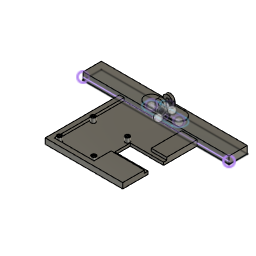
Plate (Autodesk Fusion 360 design; units mm, degrees)
Autodesk Fusion 360 part; units mm, degrees
sketch "스케치3" plane through (0, 0, 0) normal (0, 0, 1) x (1, 0, 0)
  line L0 (-80, 10) -> (80, 10)
  line L1 (80, 10) -> (80, -10)
  line L2 (80, -10) -> (-80, -10)
  line L3 (-80, -10) -> (-80, 10)
  dimension "d22" = 20
  dimension "d23" = 160
  dimension "d24" = 80
  dimension "d25" = 10
  constraint horizontal L0
  constraint vertical L1
  constraint horizontal L2
  constraint vertical L3
  measures "d22" distance of L0.end L1.end
  measures "d23" distance of L0.start L0.end
  measures "d24" distance of origin L1
  measures "d25" distance of origin L0
extrude "돌출3" add sketch "스케치3" along normal blind 3 and the other way blind 5
sketch "스케치4" plane through (0, 0, 3) normal (0, 0, 1) x (-1, 0, 0)
  arc A0 (-15, 7.5) -> (-15, -7.5) centre (-15, 0) ccw
  line L0 (0, 7.5) -> (-15, 7.5)
  line L1 (-15, -7.5) -> (0, -7.5)
  line L2 (80, 10) -> (-80, 10)
  line L3 (0, 7.5) -> (15, 7.5)
  arc A1 (15, -7.5) -> (15, 7.5) centre (15, 0) ccw
  line L4 (15, -7.5) -> (0, -7.5)
  dimension "d43" = 15
  measures "d43" distance of L0.start L1.end
extrude "돌출4" add sketch "스케치4" along normal blind 1
sketch "스케치6" plane through (0, 0, 0) normal (0, 1, 0) x (1, 0, 0)
  line L0 (-15, -4) -> (15, -4)
  line L1 (0, -4) -> (5, -4)
  line L2 (5, -4) -> (5, -10)
  line L3 (0, -4) -> (-3, -4)
  line L4 (-5, -10) -> (-5, -4)
  arc A0 (-5, -10) -> (5, -10) centre (0, -10) ccw
  line L5 (5, -4) -> (-5, -4)
  dimension "d34" = 5
  dimension "d68" = 6
  constraint midpoint L0 L1.start
  constraint parallel L0 L1
  constraint perpendicular L1 L2
  constraint coincident L0 L3.end
  constraint tangent L2 A0
  constraint coincident L0 L4.end
  constraint tangent L4 A0
  constraint perpendicular L0 L4
  measures "d34" distance of L1.start L1.end
  measures "d68" distance of L4.start L4.end
extrude "돌출5" add sketch "스케치6" along normal blind 3 from surface at 2.5
extrude "돌출6" add 1 faces at (1.6667, 2.5, 8) along direction (0, -1, 0) blind 3 from surface at 5.5
sketch "스케치7" plane through (0, 5.5, 0) normal (0, 1, 0) x (-1, 0, 0)
  circle A0 centre (0, 10) radius 1.7
  point P0 (0, 10)
  dimension "d41" = 3.4
  constraint coincident P0 A0.centre
  measures "d41" diameter of A0
extrude "돌출7" cut sketch "스케치7" against normal through all
move_body "이동1" bodies 1 to x (1, 0, 0) y (0, 1, 0) z (0, 0, 1) at (0, 0, 5)
sketch "스케치9" plane through (0, 0, 0) normal (0, 0, 1) x (1, 0, 0)
  line L0 (-80, -10) -> (80, -10)
  line L1 (-35, -10) -> (-35, -86.6)
  line L2 (-35, -86.6) -> (40, -86.6)
  line L3 (40, -86.6) -> (40, -10)
  line L4 (-35, -10) -> (40, -10)
  line L5 (-35, -10) -> (8.3, -10)
  line L6 (40, -67.8) -> (8.5, -67.8)
  line L7 (8.5, -67.8) -> (8.5, -86.6)
  line L8 (40, -43.3) -> (28, -43.3)
  line L9 (28, -43.3) -> (28, -10)
  dimension "d46" = 76.6
  dimension "d47" = 75
  dimension "d69" = 31.5
  dimension "d70" = 57.8
  dimension "d75" = 12
  dimension "d76" = 33.3
  constraint coincident L0 L1.start
  constraint perpendicular L0 L1
  constraint perpendicular L1 L2
  constraint coincident L0 L3.end
  constraint perpendicular L0 L3
  constraint perpendicular L1 L5
  constraint coincident L3 L6.start
  constraint perpendicular L3 L6
  constraint coincident L2 L7.end
  constraint perpendicular L2 L7
  constraint coincident L3 L8.start
  constraint perpendicular L3 L8
  constraint perpendicular L0 L9
  constraint coincident L0 L9.end
  measures "d46" distance of L1.start L1.end
  measures "d47" distance of L1.end L2.end
  measures "d69" distance of L6.start L6.end
  measures "d70" distance of L3.end L6.start
  measures "d75" distance of L8.start L8.end
  measures "d76" distance of L8.end L9.end
extrude "돌출8" add sketch "스케치9" along normal blind 3
sketch "스케치10" plane through (0, 0, 0) normal (0, 0, 1) x (1, 0, 0)
  line L0 (-40, -10) -> (-40, -91.6)
  line L1 (-40, -91.6) -> (45, -91.6)
  line L2 (45, -91.6) -> (45, -10)
  line L3 (-35, -10) -> (-35, -86.6)
  line L4 (-35, -86.6) -> (40, -86.6)
  line L5 (40, -86.6) -> (40, -10)
  line L6 (-35, -10) -> (-80, -10)
  line L7 (80, -10) -> (40, -10)
  dimension "d57" = 5
  dimension "d58" = 5
  dimension "d59" = 5
  constraint vertical L0
  constraint perpendicular L0 L1
  constraint perpendicular L1 L2
  constraint coincident L0.start L6
  constraint coincident L2.end L7
  measures "d57" distance of L0 L3
  measures "d58" distance of L1 L4
  measures "d59" distance of L2 L5
extrude "돌출9" add sketch "스케치10" sketch "스케치9" along normal blind 6 of sketch 2 contours L0 L3 L4 L8 L9 | L2 L3 L6 L7
sketch "스케치11" plane through (45, 0, 0) normal (1, 0, 0) x (0, 1, 0)
  line L0 (-86.6, 6) -> (-10, 6)
  line L1 (-10, 0) -> (-91.6, 0)
  line L2 (-67.8, 8) -> (-43.3, 8)
  line L3 (-43.3, 8) -> (-43.3, 3)
  line L4 (-43.3, 3) -> (-67.8, 3)
  line L5 (-67.8, 3) -> (-67.8, 8)
  point P0 (-67.8, 3)
  point P1 (-67.8, 6)
  point P2 (-43.3, 6)
  point P3 (-43.3, 3)
  dimension "d71" = 24.5
  dimension "d72" = 5
  constraint parallel L0 L2
  constraint perpendicular L2 L3
  constraint coincident P0 L4.end
  measures "d71" distance of L2.start L2.end
  measures "d72" distance of L2.end P3
extrude "돌출12" cut sketch "스케치11" against normal blind 5 contours L0 L3 L4 L5
sketch "스케치12" plane through (0, 0, 3) normal (0, 0, 1) x (-1, 0, 0)
  circle A0 centre (32.2, 83.8) radius 2.5
  line L0 (-8.5, 86.6) -> (35, 86.6)
  line L1 (35, 86.6) -> (35, 10)
  circle A1 centre (-5.5, 83.8) radius 2.5
  circle A2 centre (32.2, 46.8) radius 2.5
  circle A3 centre (-5.5, 46.8) radius 2.5
  dimension "d77" = 5
  dimension "d78" = 2.8
  dimension "d79" = 2.8
  dimension "d80" = 5
  dimension "d81" = 37.7
  dimension "d82" = 5
  dimension "d83" = 37
  dimension "d84" = 5
  measures "d77" diameter of A0
  measures "d78" distance of A0.centre L0
  measures "d79" distance of A0.centre L1
  measures "d80" diameter of A1
  measures "d81" distance of A0.centre A1.centre
  measures "d82" diameter of A2
  measures "d83" distance of A0.centre A2.centre
  measures "d84" diameter of A3
extrude "돌출13" add sketch "스케치12" along normal blind 5
sketch "스케치13" plane through (0, 0, 8) normal (0, 0, 1) x (-1, 0, 0)
  circle A0 centre (32.2, 46.8) radius 1.8
  circle A1 centre (32.2, 46.8) radius 2.5
  circle A2 centre (-5.5, 46.8) radius 1.8
  circle A3 centre (-5.5, 46.8) radius 2.5
  circle A4 centre (-5.5, 83.8) radius 1.8
  circle A5 centre (-5.5, 83.8) radius 2.5
  circle A6 centre (32.2, 83.8) radius 1.8
  circle A7 centre (32.2, 83.8) radius 2.5
  dimension "d87" = 3.6
  dimension "d88" = 3.6
  dimension "d89" = 3.6
  dimension "d90" = 3.6
  constraint concentric A0 A1
  constraint concentric A2 A3
  constraint concentric A4 A5
  constraint concentric A6 A7
  measures "d87" diameter of A0
  measures "d88" diameter of A2
  measures "d89" diameter of A4
  measures "d90" diameter of A6
extrude "돌출14" cut sketch "스케치13" against normal blind 1 contours A0 | A2 | A4 | A6
sketch "스케치14" plane through (0, 0, 7) normal (0, 0, 1) x (-1, 0, 0)
  circle A0 centre (32.2, 46.8) radius 1.25
  circle A1 centre (32.2, 46.8) radius 2.5
  circle A2 centre (-5.5, 46.8) radius 1.25
  circle A3 centre (-5.5, 46.8) radius 2.5
  circle A4 centre (-5.5, 83.8) radius 1.25
  circle A5 centre (-5.5, 83.8) radius 2.5
  circle A6 centre (32.2, 83.8) radius 1.25
  circle A7 centre (32.2, 83.8) radius 2.5
  dimension "d93" = 2.5
  dimension "d94" = 2.5
  dimension "d95" = 2.5
  dimension "d96" = 2.5
  constraint concentric A0 A1
  constraint concentric A2 A3
  constraint concentric A4 A5
  constraint concentric A6 A7
  measures "d93" diameter of A0
  measures "d94" diameter of A2
  measures "d95" diameter of A4
  measures "d96" diameter of A6
extrude "돌출15" cut sketch "스케치14" against normal blind 2 contours A0 | A2 | A4 | A6
sketch "스케치15" plane through (0, 0, 3) normal (0, 0, 1) x (-1, 0, 0)
  line L0 (-45, 63.8) -> (-8.5, 63.8)
  line L1 (-8.5, 63.8) -> (-8.5, 46.8)
  line L2 (-8.5, 46.8) -> (-45, 46.8)
  line L3 (-45, 46.8) -> (-45, 63.8)
  line L4 (-45, 43.3) -> (-45, 67.8)
  line L5 (-8.5, 67.8) -> (-8.5, 86.6)
  dimension "d99" = 17
  constraint horizontal L0
  constraint vertical L1
  constraint horizontal L2
  constraint vertical L3
  constraint coincident L0.start L4
  constraint collinear L1 L5
  measures "d99" distance of L0.start L2.end
extrude "돌출16" cut sketch "스케치15" against normal through all
equation "d46 = 43.3 mm + 33.3 mm"
